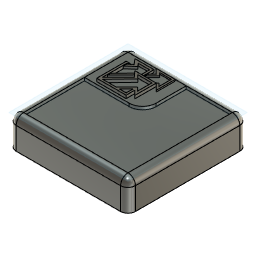
Magnet logo FWR v3 (Autodesk Fusion 360 design; units mm, degrees)
Autodesk Fusion 360 part; units mm, degrees
note: some values were not read from the file. Set by a fixed rule: which sketch regions a step uses.
sketch "Sketch1" plane through (0, 0, 0) normal (0, 0, 1) x (1, 0, 0)
  line L0 (0, 0) -> (40, 0)
  line L1 (40, 0) -> (40, 40)
  line L2 (40, 40) -> (0, 40)
  line L3 (0, 40) -> (0, 0)
  dimension "d1" = 40
  dimension "d2" = 40
  constraint horizontal L0
  constraint vertical L1
  constraint horizontal L2
  constraint vertical L3
  constraint coincident L0.start L3.end
  measures "d1" distance of L0.start L0.end
  measures "d2" distance of L0.start L2.end
extrude "Extrude1" add sketch "Sketch1" along normal blind 15 makes body 1
sketch "Sketch2" plane through (0, 0, 15) normal (0, 0, 1) x (-1, 0, 0)
  line L0 (0, -40) -> (0, 0)
  line L1 (0, 0) -> (-40, 0)
  line L2 (-40, 0) -> (-40, -40)
  line L3 (-40, -40) -> (0, -40)
fillet "Fillet1" radius 2.5 4 edges at (20, 40, 15) (40, 20, 15) (20, 0, 15) (0, 20, 15) on bodies 1
fillet "Fillet2" radius 2.5 8 edges at (0, 0, 6.25) (0.7322, 0.7322, 14.2678) (40, 0, 6.25) (39.2678, 0.7322, 14.2678) (40, 40, 6.25) (39.2678, 39.2678, 14.2678) (0, 40, 6.25) (0.7322, 39.2678, 14.2678) on bodies 1
sketch "Sketch4" plane through (0, 0, 15) normal (0, 0, 1) x (-1, 0, 0)
  line L0 (-22, -37.5) -> (-37.5, -37.5)
  line L1 (-37.5, -37.5) -> (-37.5, -22.8983)
  line L2 (-37.5, -22.8983) -> (-22, -22.8983)
  line L3 (-22, -22.8983) -> (-22, -37.5)
  line L4 (-22, -22.8983) -> (-2.5, -22.8983)
  line L5 (-2.5, -22.8983) -> (-2.5, -2.5)
  line L6 (-2.5, -2.5) -> (-22, -2.5)
  line L7 (-22, -2.5) -> (-22, -22.8983)
  line L8 (-22, -22.8983) -> (-37.5, -22.8983)
  line L9 (-37.5, -22.8983) -> (-37.5, -2.5)
  line L10 (-37.5, -2.5) -> (-22, -2.5)
  line L11 (-22, -2.5) -> (-22, -22.8983)
  constraint horizontal L0
  constraint vertical L1
  constraint horizontal L2
  constraint vertical L3
  constraint horizontal L4
  constraint vertical L5
  constraint horizontal L6
  constraint vertical L7
  constraint horizontal L8
  constraint vertical L9
  constraint horizontal L10
  constraint vertical L11
extrude "Extrude3" cut sketch "Sketch4" against normal blind 1 bodies 1
fillet "Fillet3" radius 4.5 1 edges at (22, 22.8983, 14.5) on bodies 1
ref_plane "WorkPlane1" through (20, 20, 14) normal (0, 0, 1) x (-1, 0, 0)
sketch "Sketch6" plane through (20, 20, 14) normal (0, 0, 1) x (1, 0, 0)
  line L0 (-17.5, 17.5) -> (2, 17.5)
  line L1 (2, 17.5) -> (2, 7.4)
  line L2 (-2.5, 2.9) -> (-17.5, 2.9)
  line L3 (-17.5, 2.9) -> (-17.5, 17.5)
  arc A0 (-2.5, 2.9) -> (2, 7.4) centre (-2.5, 7.4) ccw
  dimension "d23" = 4.5
  constraint horizontal L0
  constraint vertical L1
  constraint horizontal L2
  constraint vertical L3
  constraint tangent L1 A0
  constraint tangent L2 A0
  measures "d23" radius of A0
extrude "Extrude7" cut sketch "Sketch6" against normal blind 15 bodies 1
ref_plane "WorkPlane2" through (20, 20, 0) normal (0, 0, -1) x (-1, 0, 0)
sketch "Sketch7" plane through (20, 20, 0) normal (0, 0, -1) x (1, 0, 0)
  circle A0 centre (-8, -11) radius 7.5
  line L0 (-17.5, -20) -> (2, -20)
  line L1 (2, -20) -> (2, -2.9)
  line L2 (2, -2.9) -> (-20, -2.9)
  line L3 (-20, -2.9) -> (-20, -17.5)
  arc A1 (-20, -17.5) -> (-17.5, -20) centre (-17.5, -17.5) ccw
  dimension "d27" = 15
  dimension "d28" = 2.5
  constraint horizontal L0
  constraint vertical L1
  constraint horizontal L2
  constraint vertical L3
  constraint tangent L0 A1
  constraint tangent L3 A1
  measures "d27" diameter of A0
  measures "d28" radius of A1
extrude "Extrude8" add sketch "Sketch7" against normal blind 3 bodies 1
sketch "Sketch8" plane through (0, 0, 0) normal (0, 0, -1) x (1, 0, 0)
  line L0 (15.7417, -37.5) -> (8.2583, -37.5)
  arc A0 (15.7417, -37.5) -> (8.2583, -37.5) centre (12, -31) ccw
  line L1 (2.5, -40) -> (37.5, -40)
  arc A1 (37.5, -40) -> (40, -37.5) centre (37.5, -37.5) ccw
  line L2 (40, -37.5) -> (40, -2.5)
  arc A2 (40, -2.5) -> (37.5, 0) centre (37.5, -2.5) ccw
  line L3 (37.5, 0) -> (2.5, 0)
  arc A3 (2.5, 0) -> (0, -2.5) centre (2.5, -2.5) ccw
  line L4 (0, -2.5) -> (0, -37.5)
  arc A4 (0, -37.5) -> (2.5, -40) centre (2.5, -37.5) ccw
  circle A5 centre (12, -31) radius 7.5
  constraint concentric A0 A5
extrude "Extrude9" cut sketch "Sketch8" against normal blind 3 contours L0 A5 | L0 A0 A5 bodies 1
sketch "Sketch9" plane through (0, 0, 3) normal (0, 0, 1) x (-1, 0, 0)
  line L0 (-8.2583, -37.5) -> (-2.5, -37.5)
  line L1 (-2.5, -37.5) -> (-2.5, -22.9)
  line L2 (-2.5, -22.9) -> (-17.5, -22.9)
  arc A0 (-17.5, -22.9) -> (-22, -27.4) centre (-17.5, -27.4) ccw
  line L3 (-22, -27.4) -> (-22, -37.5)
  line L4 (-22, -37.5) -> (-15.7417, -37.5)
  arc A1 (-8.2583, -37.5) -> (-15.7417, -37.5) centre (-12, -31) ccw
  line L5 (-22, -38.6854) -> (-2.5, -38.6854)
  line L6 (-2.5, -38.6854) -> (-2.5, -22.9)
  line L7 (-2.5, -22.9) -> (-22, -22.9)
  line L8 (-22, -22.9) -> (-22, -38.6854)
  constraint horizontal L5
  constraint vertical L6
  constraint horizontal L7
  constraint vertical L8
  constraint coincident L1.end L2.start
extrude "Extrude10" add sketch "Sketch9" along normal blind 10.5 contours L0 L1 L2 A0 L3 L4 A1 L6 L7 L8 | L0 L4 A1 L5 L6 L8 bodies 1
sketch "Sketch10" plane through (0, 0, 15) normal (0, 0, 1) x (-1, 0, 0)
sketch "Sketch11" plane through (0, 0, 15) normal (0, 0, 1) x (-1, 0, 0)
  line L0 (-7.2, -33.6) -> (-5.8, -33.6)
  line L1 (-5.8, -33.6) -> (-5.8, -23.7036)
  line L2 (-5.8, -23.7036) -> (-15.65, -23.7036)
  line L3 (-15.65, -23.7036) -> (-15.65, -26.6)
  line L4 (-14.9808, -26.7074) -> (-14.9808, -24.4)
  line L5 (-14.9808, -24.4) -> (-6.5, -24.4)
  line L6 (-6.5, -24.4) -> (-6.5, -33)
  line L7 (-6.5, -33) -> (-7.2, -33.6)
  line L8 (-7.2, -33.6) -> (-7.8738, -34.1775)
  line L9 (-7.8738, -34.1775) -> (-6.3153, -35.9958)
  line L10 (-6.3153, -35.9958) -> (-12.7231, -35.9958)
  line L11 (-12.7231, -35.9958) -> (-12.7231, -32.2825)
  line L12 (-12, -32.2825) -> (-12, -35.2233)
  line L13 (-12, -35.2233) -> (-8.2, -35.2233)
  line L14 (-8.2, -35.2233) -> (-9.1, -34.2)
  line L15 (-9.1, -34.2) -> (-6.5, -31.9)
  line L16 (-6.5, -27.7029) -> (-10.4908, -31.7447)
  line L17 (-10.9818, -31.2068) -> (-6.5, -26.6461)
  line L18 (-12.7231, -33.9853) -> (-14.0767, -35.3627)
  line L19 (-14.0767, -35.3627) -> (-12.3664, -37.0433)
  line L20 (-12.3664, -37.0433) -> (-18.7932, -37.0433)
  line L21 (-18.7932, -37.0433) -> (-18.7932, -30.7)
  line L22 (-18.7932, -30.7) -> (-17.2111, -32.2825)
  line L23 (-17.1601, -33.2423) -> (-18.1196, -32.2825)
  line L24 (-18.1196, -32.2825) -> (-18.1196, -36.4)
  line L25 (-18.1196, -36.4) -> (-14.2, -36.4)
  line L26 (-14.2, -36.4) -> (-15.1573, -35.4424)
  line L27 (-15.1573, -35.4424) -> (-12.7231, -33.009)
  line L28 (-6.5, -25) -> (-11.8057, -30.3041)
  line L29 (-17.2111, -32.2825) -> (-10, -32.2825)
  line L30 (-10, -32.2825) -> (-11.8057, -30.3041)
  line L31 (-7.1, -24.4) -> (-12.9, -30.4)
  line L32 (-12.9, -30.4) -> (-11.6409, -31.6171)
  line L33 (-11.6409, -31.6171) -> (-16.4, -31.6171)
  line L34 (-16.4, -31.6171) -> (-16.4, -26.8366)
  line L35 (-15.1966, -28.0333) -> (-11.6, -24.4)
  line L36 (-12.7, -24.4) -> (-14.9808, -26.7074)
  line L37 (-15.65, -26.6) -> (-17.1628, -25.0956)
  line L38 (-17.1628, -25.0956) -> (-17.2111, -32.2825)
  line L39 (-15.1966, -28.0333) -> (-16.4, -26.8366)
  line L40 (-17.1601, -33.2423) -> (-16.1399, -32.2825)
  constraint horizontal L0
  constraint perpendicular L0 L1
  constraint perpendicular L1 L2
  constraint perpendicular L2 L3
  constraint parallel L3 L4
  constraint perpendicular L4 L5
  constraint perpendicular L5 L6
  constraint parallel L7 L8
  constraint perpendicular L8 L9
  constraint parallel L0 L10
  constraint perpendicular L10 L11
  constraint perpendicular L12 L13
  constraint coincident L6 L15.end
  constraint coincident L6 L16.start
  constraint coincident L6 L17.end
  constraint coincident L11 L18.start
  constraint parallel L17 L18
  constraint perpendicular L18 L19
  constraint perpendicular L11 L20
  constraint perpendicular L20 L21
  constraint parallel L21 L24
  constraint perpendicular L24 L25
  constraint coincident L11 L27.end
  constraint perpendicular L26 L27
  constraint coincident L6 L28.start
  constraint parallel L27 L28
  constraint horizontal L29
  constraint coincident L16.end L30
  constraint coincident L17.start L30
  constraint coincident L12.start L29
  constraint perpendicular L12 L29
  constraint coincident L11.end L29
  constraint coincident L5 L31.start
  constraint perpendicular L31 L32
  constraint parallel L5 L33
  constraint perpendicular L33 L34
  constraint coincident L5 L35.end
  constraint coincident L5 L36.start
  constraint parallel L37 L39
  constraint coincident L29 L40.end
extrude "Extrude11" add sketch "Sketch11" along normal blind 1 separate body contours L0 L1 L2 L3 L6 L7 L28 L29 L30 L37 L38 makes body 2
extrude "Extrude13" add sketch "Sketch11" along normal blind 0.3 contours L6 L7 L8 L9 L10 L11 L12 L13 L14 L15 L29 | L6 L16 L17 L30 bodies 2 1
extrude "Extrude15" add sketch "Sketch11" along normal blind 0.5 separate body contours L11 L18 L19 L20 L21 L22 L23 L24 L25 L26 L27 L29 L40 makes body 3
extrude "Extrude16" add 1 faces at (7.463, 35.1322, 15.3) along direction (0, 0, 1) blind 0.5 on bodies 2 bodies 2 3
extrude "Extrude17" add 1 faces at (7.9939, 28.5186, 15.3) along direction (0, 0, 1) blind 0.5 on bodies 2 bodies 2
extrude "Extrude18" cut 1 faces at (18.2437, 8.005, 0) along direction (0, 0, 1) blind 5 on bodies 2 bodies 2
extrude "Extrude19" cut 1 faces at (14.4726, 31.3694, 3) along direction (0, 0, 1) blind 5 on bodies 2 bodies 2
sketch "Sketch12" plane through (0, 0, 0) normal (0, 0, 1) x (1, 0, 0)
